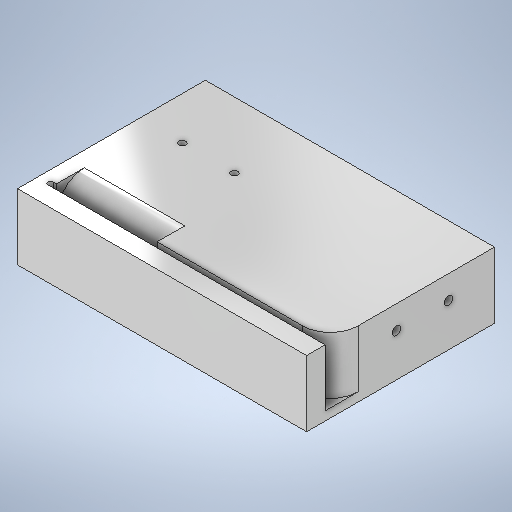
# Autodesk Inventor part: Tamale Assembly Plate FLEX V1 Print Section
Saved by Autodesk Inventor 2025 (Build 290162000, 162)
## iProperties
Created: 2022-03-23
Part Number: Tamale Assembly Plate FLEX V1 Print Section
Material: Generic
Document SubType Name: Modeling
Designer: Caleb
Density: 1 g/cm^3
Appearance: Aluminum - Dark
Author: Caleb
Autodesk Inventor part; units mm, degrees
ref_plane "YZ Plane" through (0, 0, 0) normal (1, 0, 0) x (0, 1, 0)
ref_plane "XZ Plane" through (0, 0, 0) normal (0, 1, 0) x (-1, 0, 0)
ref_plane "XY Plane" through (0, 0, 0) normal (0, 0, 1) x (1, 0, 0)
sketch "Sketch1" plane through (0, 0, 0) normal (0, 1, 0) x (-1, 0, 0)
  line L0 (-63.5, -111) -> (63.5, -111)
  line L1 (63.5, -111) -> (63.5, 111)
  line L2 (63.5, 111) -> (-63.5, 111)
  line L3 (-63.5, 111) -> (-63.5, -111)
  line L4 (-63.5, -111) -> (63.5, 111) construction
  line L5 (63.5, -111) -> (-63.5, 111) construction
  point P0 (0, 0)
  dimension "d0" = 127
  dimension "d1" = 222
  constraints: 12 end point, 2 midpoint, 2 parallel, 1 horizontal, 1 perpendicular
  measures "d0" distance of L2.end L1.end
  measures "d1" distance of L1.end L0.end
extrude "Extrusion1" add sketch "Sketch1" along normal blind 19.05
sketch "Sketch12" plane through (0, 19.05, 0) normal (0, 1, 0) x (1, 0, 0)
  line L0 (63.5, -111) -> (63.5, 111) projected
  line L1 (-16.5, -104.15) -> (63.5, -104.15)
  line L2 (63.5, -104.15) -> (63.5, -105.65)
  line L3 (63.5, -105.65) -> (-16.5, -105.65)
  circle A0 centre (33, -60.25) radius 1.2295 projected
  circle A1 centre (33, -47.45) radius 1.2295 projected
  arc A2 (-16.5, -104.15) -> (-16.5, -105.65) centre (-16.5, -104.9) ccw
  circle A3 centre (-33, -9.45) radius 1.2295 projected
  circle A4 centre (-33, -60.25) radius 1.2295 projected
  circle A5 centre (33, -98.25) radius 1.2295 projected
  line L4 (-16.5, -53.35) -> (63.5, -53.35)
  line L5 (63.5, -53.35) -> (63.5, -54.85)
  line L6 (63.5, -54.85) -> (-16.5, -54.85)
  arc A6 (-16.5, -53.35) -> (-16.5, -54.85) centre (-16.5, -54.1) ccw
  line L7 (-16.5, -2.55) -> (63.5, -2.55)
  line L8 (63.5, -2.55) -> (63.5, -4.05)
  line L9 (63.5, -4.05) -> (-16.5, -4.05)
  arc A7 (-16.5, -2.55) -> (-16.5, -4.05) centre (-16.5, -3.3) ccw
  line L10 (-16.5, 48.25) -> (63.5, 48.25)
  line L11 (63.5, 48.25) -> (63.5, 46.75)
  line L12 (63.5, 46.75) -> (-16.5, 46.75)
  arc A8 (-16.5, 48.25) -> (-16.5, 46.75) centre (-16.5, 47.5) ccw
  point P0 (0, 0)
  point P1 (63.5, -60.2)
  point P2 (63.5, -9.4)
  point P3 (63.5, 41.4)
  dimension "d156" = 1.5
  dimension "d157" = 12.8
  dimension "d159" = 0.75
  dimension "d160" = 80
  dimension "d161" = 50.8
  dimension "d162" = 5.9
  dimension "d165" = 50.8
  constraints: 24 end point, 8 point on circle, 4 centre point, 1 horizontal, 1 parallel, 1 perpendicular, 1 point on line, 1 vertical, 1 vertical alignment, 30 other
  measures "d156" distance of L3.end L1.start
  measures "d157" distance of A0.centre A1.centre
  measures "d159" radius of A2
  measures "d160" distance from line of L0 A2.centre
  measures "d161" distance of A3.centre A4.centre
  measures "d162" distance from line of L1 A5.centre
  measures "d165" distance of L1.start L4.start
extrude "Extrusion7" cut sketch "Sketch12" against normal blind 16.5 contours L3 A2 L1 L0 | L6 A6 L4 L0 | L9 A7 L7 L0 | L12 A8 L10 L0
sketch "Sketch13" plane through (63.5, 0, 111) normal (1, 0, 0) x (0, 0, -1)
  line L0 (0, 0) -> (222, 0) projected
  line L1 (0, 0) -> (0, 19.05) projected
  line L2 (56.15, 2.55) -> (56.15, 19.05) projected
  line L3 (5.35, 2.55) -> (5.35, 19.05) projected
  point P0 (111, 0)
  point P1 (25.91, 12.3)
  point P2 (40.91, 12.3)
  point P3 (0, 17.05)
  point P4 (56.65, 17.05)
  point P5 (5.85, 17.05)
  point P6 (76.71, 12.3)
  point P7 (91.71, 12.3)
  point P8 (127.51, 12.3)
  point P9 (142.51, 12.3)
  point P10 (178.31, 12.3)
  point P11 (193.31, 12.3)
  point P12 (56.15, 19.05)
  point P13 (5.35, 19.05)
  dimension "d176" = 50.8
  dimension "d173" = 12.3
  dimension "d174" = 15
  dimension "d175" = 25.91
  dimension "d179" = 50.8
  constraints: 1 horizontal, 1 horizontal alignment, 8 other
  measures "d173" distance from line of L0 point (25.91, 12.3)
  measures "d174" distance of point (25.91, 12.3) point (40.91, 12.3)
  measures "d175" distance from line of L1 point (25.91, 12.3)
  measures "d179" distance of point (25.91, 12.3) point (76.71, 12.3)
hole "Hole7" at (63.5, 12.3, 85.09) at (63.5, 12.3, 70.09) at (63.5, 12.3, 34.29) at (63.5, 12.3, 19.29) at (63.5, 12.3, -16.51) at (63.5, 12.3, -31.51) at (63.5, 12.3, -67.31) at (63.5, 12.3, -82.31) direction (-1, 0, 0) diameter 2.459 depth 8.8 tip angle 118 thread size "M3x0.5" class "6H" standard "ANSI Metric M Profile"
sketch "Sketch14" plane through (63.5, 0, 111) normal (1, 0, 0) x (0, 0, -1)
  line L0 (6.85, 19.05) -> (6.85, 2.55) projected
  arc A0 (14.85, 19.05) -> (6.85, 11.05) centre (14.85, 11.05) ccw
  line L1 (14.85, 11.05) -> (14.85, 19.05) construction
  line L2 (14.85, 11.05) -> (6.85, 11.05) construction
  line L3 (6.85, 19.05) -> (56.15, 19.05) projected
  line L4 (14.85, 19.05) -> (6.85, 19.05)
  line L5 (6.85, 19.05) -> (6.85, 11.05)
  arc A1 (65.65, 19.05) -> (57.65, 11.05) centre (65.65, 11.05) ccw
  line L6 (65.65, 19.05) -> (57.65, 19.05)
  line L7 (57.65, 19.05) -> (57.65, 11.05)
  arc A2 (116.45, 19.05) -> (108.45, 11.05) centre (116.45, 11.05) ccw
  line L8 (116.45, 19.05) -> (108.45, 19.05)
  line L9 (108.45, 19.05) -> (108.45, 11.05)
  arc A3 (167.25, 19.05) -> (159.25, 11.05) centre (167.25, 11.05) ccw
  line L10 (167.25, 19.05) -> (159.25, 19.05)
  line L11 (159.25, 19.05) -> (159.25, 11.05)
  point P0 (111, 0)
  dimension "d191" = 90
  dimension "d192" = 8
  dimension "d193" = 8
  dimension "d198" = 50.8
  constraints: 20 end point, 8 point on circle, 4 centre point, 1 horizontal, 1 horizontal alignment, 1 perpendicular, 1 point on line, 21 other
  measures "d191" angle of L1 L2
  measures "d192" distance from line of L3 L1.start
  measures "d193" distance from line of L0 L1.start
  measures "d198" distance of L1.start A1.centre
extrude "Extrusion8" cut sketch "Sketch14" against normal blind 79
extrude "Extrusion10" add sketch "Sketch14" against normal blind 50
sketch "Sketch15" plane through (0, 19.05, 0) normal (0, 1, 0) x (1, 0, 0)
  arc A0 (55.5, -104.15) -> (63.5, -96.15) centre (55.5, -96.15) ccw
  line L0 (55.5, -96.15) -> (55.5, -104.15) construction
  line L1 (55.5, -96.15) -> (63.5, -96.15) construction
  line L2 (-15.5, -104.15) -> (63.5, -104.15) projected
  line L3 (63.5, -96.15) -> (63.5, -54.85) projected
  line L4 (-16.5, -104.15) -> (63.5, -104.15) projected
  line L5 (55.5, -104.15) -> (63.5, -104.15)
  line L6 (63.5, -104.15) -> (63.5, -96.15)
  arc A1 (55.5, -53.35) -> (63.5, -45.35) centre (55.5, -45.35) ccw
  line L7 (63.5, -53.35) -> (63.5, -45.35)
  line L8 (55.5, -53.35) -> (63.5, -53.35)
  arc A2 (55.5, -2.55) -> (63.5, 5.45) centre (55.5, 5.45) ccw
  line L9 (63.5, -2.55) -> (63.5, 5.45)
  line L10 (55.5, -2.55) -> (63.5, -2.55)
  arc A3 (55.5, 48.25) -> (63.5, 56.25) centre (55.5, 56.25) ccw
  line L11 (63.5, 48.25) -> (63.5, 56.25)
  line L12 (55.5, 48.25) -> (63.5, 48.25)
  point P0 (0, 0)
  point P1 (63.5, 56.25)
  point P2 (63.5, 5.45)
  dimension "d203" = 90
  dimension "d204" = 8
  dimension "d207" = 50.8
  constraints: 20 end point, 8 point on circle, 4 centre point, 2 point on line, 1 collinear, 1 perpendicular, 1 tangent, 1 vertical, 24 other
  measures "d203" angle of L0 L1
  measures "d204" distance of L0.start L1.end
  measures "d207" distance of L0.start A1.centre
extrude "Extrusion9" cut sketch "Sketch15" against normal up to surface (16.5 mm away)
sketch "Sketch16" plane through (0, 19.05, 0) normal (0, 1, 0) x (1, 0, 0)
  line L0 (-15.5, -96.15) -> (13.5, -96.15) projected
  line L1 (13.5, -104.15) -> (13.5, -96.15) projected
  point P0 (0, 0)
  point P1 (7.5, -75.85)
  point P2 (-7.5, -75.85)
  point P3 (-16.5, -96.15)
  point P4 (-7.5, -25.05)
  point P5 (7.5, -25.05)
  point P6 (-7.5, 25.75)
  point P7 (7.5, 25.75)
  point P8 (-7.5, 76.55)
  point P9 (7.5, 76.55)
  dimension "d216" = 20.3
  dimension "d217" = 15
  dimension "d218" = 6
  dimension "d221" = 50.8
  constraints: 1 horizontal alignment, 1 vertical, 6 other
  measures "d216" distance from line of point (7.5, -75.85) L0
  measures "d217" distance of point (-7.5, -75.85) point (7.5, -75.85)
  measures "d218" distance from line of L1 point (7.5, -75.85)
  measures "d221" distance of point (-7.5, -75.85) point (-7.5, -25.05)
hole "Hole8" at (-7.5, 19.05, 25.05) at (-7.5, 19.05, -25.75) at (7.5, 19.05, -25.75) at (-7.5, 19.05, -76.55) at (7.5, 19.05, -76.55) at (7.5, 19.05, 75.85) at (-7.5, 19.05, 75.85) at (7.5, 19.05, 25.05) direction (0, -1, 0) diameter 2 end through all
sketch "Sketch17" plane through (0, 19.05, 0) normal (0, 1, 0) x (1, 0, 0)
  line L0 (63.5, -111) -> (63.5, 111) projected
  line L1 (63.5, -111) -> (-19.9113, -111)
  line L2 (-19.9113, -111) -> (-19.9113, -56.7947)
  line L3 (-19.9113, -56.7947) -> (63.5, -56.7947)
  line L4 (63.5, -56.7947) -> (63.5, -111)
  line L5 (-63.5, 111) -> (-63.5, -111) projected
  line L6 (-19.9113, -111) -> (-63.5, -111)
  line L7 (-63.5, -111) -> (-63.5, 111)
  line L8 (-63.5, 111) -> (63.5, 111)
  point P0 (0, 0)
  constraints: 14 end point, 4 perpendicular, 2 parallel, 1 horizontal
extrude "Extrusion11" cut sketch "Sketch17" against normal through all contours L3 L2 L6 L5 L8 L0
body "Solid1"
